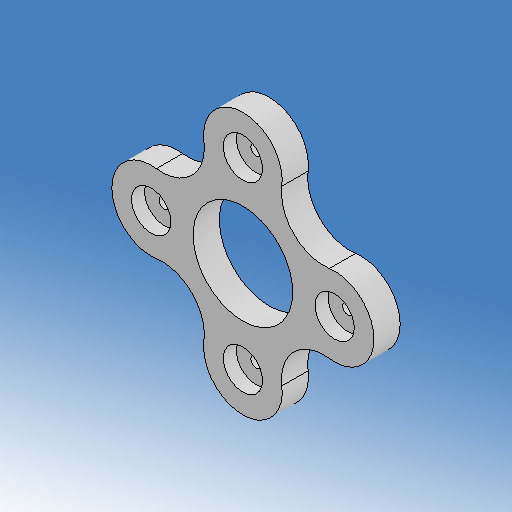
# Autodesk Inventor part: drive sprocket flange socket
Saved by Autodesk Inventor 2025 (Build 290162000, 162)
## iProperties
Created: 2023-04-05
Part Number: drive sprocket flange socket
Material: Generic
Document SubType Name: Modeling
Designer: ralph
Density: 1 g/cm^3
Appearance: Default
Author: ralph
Autodesk Inventor part; units mm, degrees
ref_plane "YZ Plane" through (0, 0, 0) normal (1, 0, 0) x (0, 1, 0)
ref_plane "XZ Plane" through (0, 0, 0) normal (0, 1, 0) x (-1, 0, 0)
sketch "Sketch1" plane through (0, 0, 0) normal (0, 0, 1) x (1, 0, 0)
  circle A0 centre (0, -8) radius 12.065 projected
  arc A1 (-7.912, -62.1223) -> (-4.7827, -62.4881) centre (0, -8) ccw projected
  arc A2 (-3.3911, -60.1215) -> (-4.7827, -62.4881) centre (5.3956, -66.8807) ccw projected
  arc A3 (3.3911, -60.1215) -> (-3.3911, -60.1215) centre (0, -62.6976) ccw projected
  arc A4 (4.7827, -62.4881) -> (3.3911, -60.1215) centre (-5.3956, -66.8807) ccw projected
  arc A5 (4.7827, -62.4881) -> (7.912, -62.1223) centre (0, -8) ccw projected
  arc A6 (8.7203, -59.4986) -> (7.912, -62.1223) centre (18.829, -64.0493) ccw projected
  arc A7 (15.3198, -57.9345) -> (8.7203, -59.4986) centre (12.6141, -61.2232) ccw projected
  arc A8 (17.2196, -59.9164) -> (15.3198, -57.9345) centre (8.3287, -66.5379) ccw projected
  arc A9 (17.2196, -59.9164) -> (20.1802, -58.8388) centre (0, -8) ccw projected
  arc A10 (20.3617, -56.0994) -> (20.1802, -58.8388) centre (31.2473, -58.1962) ccw projected
  arc A11 (26.4225, -53.0555) -> (20.3617, -56.0994) centre (24.5482, -56.8795) ccw projected
  arc A12 (28.7282, -54.5458) -> (26.4225, -53.0555) centre (21.6039, -63.0393) ccw projected
  arc A13 (28.7282, -54.5458) -> (31.3605, -52.8146) centre (0, -8) ccw projected
  arc A14 (30.9053, -50.1072) -> (31.3605, -52.8146) centre (41.9811, -49.637) ccw projected
  arc A15 (36.1008, -45.7476) -> (30.9053, -50.1072) centre (35.1589, -49.9008) ccw projected
  arc A16 (38.688, -46.666) -> (36.1008, -45.7476) centre (33.7145, -56.5735) ccw projected
  arc A17 (38.688, -46.666) -> (40.8501, -44.3744) centre (0, -8) ccw projected
  arc A18 (39.7828, -41.8449) -> (40.8501, -44.3744) centre (50.4517, -38.8332) ccw projected
  arc A19 (43.8329, -36.4047) -> (39.7828, -41.8449) centre (43.8742, -40.6631) ccw projected
  arc A20 (46.5622, -36.7017) -> (43.8329, -36.4047) centre (44.0076, -47.4891) ccw projected
  arc A21 (46.5622, -36.7017) -> (48.1375, -33.9732) centre (0, -8) ccw projected
  arc A22 (46.5156, -31.7581) -> (48.1375, -33.9732) centre (56.2023, -26.3671) ccw projected
  arc A23 (49.2019, -25.5305) -> (46.5156, -31.7581) centre (50.2242, -29.6646) ccw projected
  arc A24 (51.9262, -25.19) -> (49.2019, -25.5305) centre (51.9282, -36.2758) ccw projected
  arc A25 (51.9262, -25.19) -> (52.8298, -22.1718) centre (0, -8) ccw projected
  arc A26 (50.7408, -20.3904) -> (52.8298, -22.1718) centre (58.9232, -12.9109) ccw projected
  arc A27 (51.9185, -13.7112) -> (50.7408, -20.3904) centre (53.8666, -17.4981) ccw projected
  arc A28 (54.4908, -12.7517) -> (51.9185, -13.7112) centre (57.0493, -23.5382) ccw projected
  arc A29 (54.4908, -12.7517) -> (54.674, -9.6064) centre (0, -8) ccw projected
  arc A30 (52.2305, -8.3548) -> (54.674, -9.6064) centre (58.4674, 0.8101) ccw projected
  arc A31 (51.8361, -1.584) -> (52.2305, -8.3548) centre (54.605, -4.8196) ccw projected
  arc A32 (54.1178, -0.0572) -> (51.8361, -1.584) centre (59.0949, -9.9629) ccw projected
  arc A33 (54.1178, -0.0572) -> (53.5707, 3.0455) centre (0, -8) ccw projected
  arc A34 (50.9044, 3.6999) -> (53.5707, 3.0455) centre (54.8597, 14.0561) ccw projected
  arc A35 (48.9593, 10.1973) -> (50.9044, 3.6999) centre (52.3997, 7.6874) ccw projected
  arc A36 (50.8273, 12.2092) -> (48.9593, 10.1973) centre (57.9546, 3.7182) ccw projected
  arc A37 (50.8273, 12.2092) -> (49.5794, 15.1021) centre (0, -8) ccw projected
  arc A38 (46.8341, 15.1239) -> (49.5794, 15.1021) centre (48.2944, 26.1131) ccw projected
  arc A39 (43.443, 20.9975) -> (46.8341, 15.1239) centre (47.3695, 19.3488) ccw projected
  arc A40 (44.7967, 23.386) -> (43.443, 20.9975) centre (53.69, 16.7676) ccw projected
  arc A41 (44.7967, 23.386) -> (42.9153, 25.9131) centre (0, -8) ccw projected
  arc A42 (40.2389, 25.3013) -> (42.9153, 25.9131) centre (39.1256, 36.331) ccw projected
  arc A43 (35.5847, 30.2346) -> (40.2389, 25.3013) centre (39.7856, 29.5357) ccw projected
  arc A44 (36.3511, 32.8708) -> (35.5847, 30.2346) centre (46.531, 28.4818) ccw projected
  arc A45 (36.3511, 32.8708) -> (33.9376, 34.896) centre (0, -8) ccw projected
  arc A46 (31.4745, 33.6834) -> (33.9376, 34.896) centre (27.8475, 44.1591) ccw projected
  arc A47 (25.808, 37.4103) -> (31.4745, 33.6834) centre (30.0568, 37.6992) ccw projected
  arc A48 (25.9458, 40.1523) -> (25.808, 37.4103) centre (36.8635, 38.2292) ccw projected
  arc A49 (25.9458, 40.1523) -> (23.1303, 41.5662) centre (0, -8) ccw projected
  arc A50 (21.0132, 39.8183) -> (23.1303, 41.5662) centre (15.0682, 49.1752) ccw projected
  arc A51 (14.64, 42.138) -> (21.0132, 39.8183) centre (18.7077, 43.3989) ccw projected
  arc A52 (14.1417, 44.8378) -> (14.64, 42.138) centre (25.2086, 45.4844) ccw projected
  arc A53 (14.1417, 44.8378) -> (11.0761, 45.5644) centre (0, -8) ccw projected
  arc A54 (9.4191, 43.3754) -> (11.0761, 45.5644) centre (1.4765, 51.109) ccw projected
  arc A55 (2.6827, 44.1627) -> (9.4191, 43.3754) centre (6.35, 46.3277) ccw projected
  arc A56 (1.5753, 46.6749) -> (2.6827, 44.1627) centre (12.1948, 49.8562) ccw projected
  arc A57 (1.5753, 46.6749) -> (-1.5753, 46.6749) centre (0, -8) ccw projected
  arc A58 (-2.6827, 44.1627) -> (-1.5753, 46.6749) centre (-12.1948, 49.8562) ccw projected
  arc A59 (-9.4191, 43.3754) -> (-2.6827, 44.1627) centre (-6.35, 46.3277) ccw projected
  arc A60 (-11.0761, 45.5644) -> (-9.4191, 43.3754) centre (-1.4765, 51.109) ccw projected
  arc A61 (-11.0761, 45.5644) -> (-14.1417, 44.8378) centre (0, -8) ccw projected
  arc A62 (-14.64, 42.138) -> (-14.1417, 44.8378) centre (-25.2086, 45.4844) ccw projected
  arc A63 (-21.0132, 39.8183) -> (-14.64, 42.138) centre (-18.7077, 43.3989) ccw projected
  arc A64 (-23.1303, 41.5662) -> (-21.0132, 39.8183) centre (-15.0682, 49.1752) ccw projected
  arc A65 (-23.1303, 41.5662) -> (-25.9458, 40.1523) centre (0, -8) ccw projected
  arc A66 (-25.808, 37.4103) -> (-25.9458, 40.1523) centre (-36.8635, 38.2292) ccw projected
  arc A67 (-31.4745, 33.6834) -> (-25.808, 37.4103) centre (-30.0568, 37.6992) ccw projected
  arc A68 (-33.9376, 34.896) -> (-31.4745, 33.6834) centre (-27.8475, 44.1591) ccw projected
  arc A69 (-33.9376, 34.896) -> (-36.3511, 32.8708) centre (0, -8) ccw projected
  arc A70 (-35.5847, 30.2346) -> (-36.3511, 32.8708) centre (-46.531, 28.4818) ccw projected
  arc A71 (-40.2389, 25.3013) -> (-35.5847, 30.2346) centre (-39.7856, 29.5357) ccw projected
  arc A72 (-42.9153, 25.9131) -> (-40.2389, 25.3013) centre (-39.1256, 36.331) ccw projected
  arc A73 (-42.9153, 25.9131) -> (-44.7967, 23.386) centre (0, -8) ccw projected
  arc A74 (-43.443, 20.9975) -> (-44.7967, 23.386) centre (-53.69, 16.7676) ccw projected
  arc A75 (-46.8341, 15.1239) -> (-43.443, 20.9975) centre (-47.3695, 19.3488) ccw projected
  arc A76 (-49.5794, 15.1021) -> (-46.8341, 15.1239) centre (-48.2944, 26.1131) ccw projected
  arc A77 (-49.5794, 15.1021) -> (-50.8273, 12.2092) centre (0, -8) ccw projected
  arc A78 (-48.9593, 10.1973) -> (-50.8273, 12.2092) centre (-57.9546, 3.7182) ccw projected
  arc A79 (-50.9044, 3.6999) -> (-48.9593, 10.1973) centre (-52.3997, 7.6874) ccw projected
  arc A80 (-53.5707, 3.0455) -> (-50.9044, 3.6999) centre (-54.8597, 14.0561) ccw projected
  arc A81 (-53.5707, 3.0455) -> (-54.1178, -0.0572) centre (0, -8) ccw projected
  arc A82 (-51.8361, -1.584) -> (-54.1178, -0.0572) centre (-59.0949, -9.9629) ccw projected
  arc A83 (-52.2305, -8.3548) -> (-51.8361, -1.584) centre (-54.605, -4.8196) ccw projected
  arc A84 (-54.674, -9.6064) -> (-52.2305, -8.3548) centre (-58.4674, 0.8101) ccw projected
  arc A85 (-54.674, -9.6064) -> (-54.4908, -12.7517) centre (0, -8) ccw projected
  arc A86 (-51.9185, -13.7112) -> (-54.4908, -12.7517) centre (-57.0493, -23.5382) ccw projected
  arc A87 (-50.7408, -20.3904) -> (-51.9185, -13.7112) centre (-53.8666, -17.4981) ccw projected
  arc A88 (-52.8298, -22.1718) -> (-50.7408, -20.3904) centre (-58.9232, -12.9109) ccw projected
  arc A89 (-52.8298, -22.1718) -> (-51.9262, -25.19) centre (0, -8) ccw projected
  arc A90 (-49.2019, -25.5305) -> (-51.9262, -25.19) centre (-51.9282, -36.2758) ccw projected
  arc A91 (-46.5156, -31.7581) -> (-49.2019, -25.5305) centre (-50.2242, -29.6646) ccw projected
  arc A92 (-48.1375, -33.9732) -> (-46.5156, -31.7581) centre (-56.2023, -26.3671) ccw projected
  arc A93 (-48.1375, -33.9732) -> (-46.5622, -36.7017) centre (0, -8) ccw projected
  arc A94 (-43.8329, -36.4047) -> (-46.5622, -36.7017) centre (-44.0076, -47.4891) ccw projected
  arc A95 (-39.7828, -41.8449) -> (-43.8329, -36.4047) centre (-43.8742, -40.6631) ccw projected
  arc A96 (-40.8501, -44.3744) -> (-39.7828, -41.8449) centre (-50.4517, -38.8332) ccw projected
  arc A97 (-40.8501, -44.3744) -> (-38.688, -46.666) centre (0, -8) ccw projected
  arc A98 (-36.1008, -45.7476) -> (-38.688, -46.666) centre (-33.7145, -56.5735) ccw projected
  arc A99 (-30.9053, -50.1072) -> (-36.1008, -45.7476) centre (-35.1589, -49.9008) ccw projected
  arc A100 (-31.3605, -52.8146) -> (-30.9053, -50.1072) centre (-41.9811, -49.637) ccw projected
  arc A101 (-31.3605, -52.8146) -> (-28.7282, -54.5458) centre (0, -8) ccw projected
  arc A102 (-26.4225, -53.0555) -> (-28.7282, -54.5458) centre (-21.6039, -63.0393) ccw projected
  arc A103 (-20.3617, -56.0994) -> (-26.4225, -53.0555) centre (-24.5482, -56.8795) ccw projected
  arc A104 (-20.1802, -58.8388) -> (-20.3617, -56.0994) centre (-31.2473, -58.1962) ccw projected
  arc A105 (-20.1802, -58.8388) -> (-17.2196, -59.9164) centre (0, -8) ccw projected
  arc A106 (-15.3198, -57.9345) -> (-17.2196, -59.9164) centre (-8.3287, -66.5379) ccw projected
  arc A107 (-8.7203, -59.4986) -> (-15.3198, -57.9345) centre (-12.6141, -61.2232) ccw projected
  arc A108 (-7.912, -62.1223) -> (-8.7203, -59.4986) centre (-18.829, -64.0493) ccw projected
  circle A109 centre (0, -8) radius 31.75
  circle A110 centre (-22.225, -8) radius 2.3812 projected
  circle A111 centre (0, 14.225) radius 2.3812 projected
  circle A112 centre (0, -30.225) radius 2.3812 projected
  circle A113 centre (22.225, -8) radius 2.3812 projected
  point P0 (0, 0)
  dimension "d0" = 63.5
  constraints: 1 centre point, 1 coincident
  measures "d0" diameter of A109
extrude "Extrusion1" add sketch "Sketch1" along normal blind 6.35 contours A109 | A110 | A111 | A112 | A113
sketch "Sketch2" plane through (0, -8, 6.35) normal (0, 0, 1) x (1, 0, 0)
  circle A0 centre (0, 0) radius 31.75 projected
  circle A1 centre (0, 0) radius 12.065 projected
  circle A2 centre (22.225, 0) radius 4.7625
  circle A3 centre (0, -22.225) radius 4.7625
  circle A4 centre (-22.225, 0) radius 4.7625
  circle A5 centre (0, 22.225) radius 1.27 projected
  circle A6 centre (0, 22.225) radius 4.7625
  circle A7 centre (-22.225, 0) radius 1.27
  circle A8 centre (0, -22.225) radius 1.27
  circle A9 centre (22.225, 0) radius 1.27
  point P0 (0, 8)
  dimension "d3" = 9.525
  dimension "d4" = 9.525
  dimension "d5" = 9.525
  dimension "d6" = 9.525
  constraints: 7 centre point, 4 coincident, 3 equal radius
  measures "d3" diameter of A2
  measures "d4" diameter of A3
  measures "d5" diameter of A4
  measures "d6" diameter of A6
ref_plane "Work Plane1" through (17.341, -12.884, 3.2549) normal (0, 0, -1) x (0, 1, 0)
extrude "Extrusion2" cut sketch "Sketch2" against normal through all contours A5 | A7 | A8 | A9
extrude "Extrusion3" cut sketch "Sketch2" against normal blind 3.175 contours A2 | A3 | A4 | A6
sketch "Sketch3" plane through (0, -8, 6.35) normal (0, 0, 1) x (1, 0, 0)
  circle A0 centre (22.225, 0) radius 4.7625 projected
  circle A1 centre (0, -22.225) radius 4.7625 projected
  circle A2 centre (-22.225, 0) radius 4.7625 projected
  circle A3 centre (0, 22.225) radius 4.7625 projected
  circle A4 centre (0, 0) radius 12.065 projected
  circle A5 centre (22.225, 0) radius 9.525
  circle A6 centre (0, -22.225) radius 9.525
  circle A7 centre (-22.225, 0) radius 9.525
  circle A8 centre (0, 22.225) radius 9.525
  circle A9 centre (0, 0) radius 17.4625
  circle A10 centre (0, 0) radius 31.75 projected
  arc A11 (20.9547, -9.4399) -> (9.4399, -20.9547) centre (19.5891, -19.5891) ccw
  arc A12 (9.4399, 20.9547) -> (20.9547, 9.4399) centre (19.5891, 19.5891) ccw
  arc A13 (-20.9547, 9.4399) -> (-9.4399, 20.9547) centre (-19.5891, 19.5891) ccw
  arc A14 (-9.4399, -20.9547) -> (-20.9547, -9.4399) centre (-19.5891, -19.5891) ccw
  point P0 (0, 8)
  point P1 (20.9547, 9.4399)
  point P2 (31.75, 0)
  point P3 (0, 31.75)
  point P4 (9.4399, 20.9547)
  point P5 (-9.4399, 20.9547)
  point P6 (-31.75, 0)
  point P7 (-20.9547, 9.4399)
  point P8 (-20.9547, -9.4399)
  point P9 (0, -31.75)
  point P10 (-9.4399, -20.9547)
  dimension "d13" = 360
  constraints: 8 point on circle, 7 centre point, 2 tangent, 1 equal radius, 27 other
extrude "Extrusion4" cut sketch "Sketch3" against normal through all contours A12 A8 A10 A5 | A5 A10 A6 A11 | A8 A13 A7 A10 | A10 A7 A14 A6
body "Solid1"
